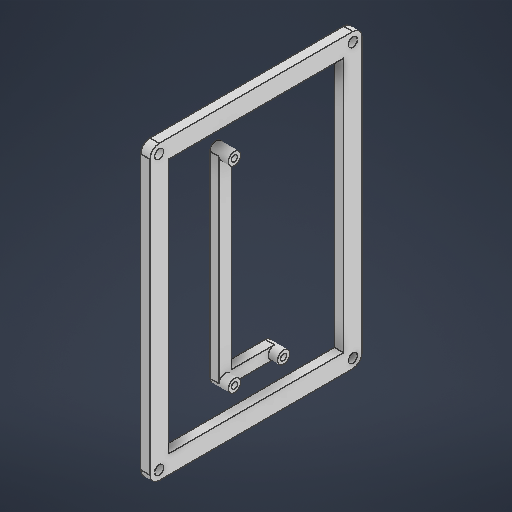
# Autodesk Inventor part: servo_drever_support
Saved by Autodesk Inventor 2026.1 (Build 301233000, 233)
## iProperties
Created: 2026-05-02
Part Number: servo_drever_support
Material: Generic
Document SubType Name: Modeling
Designer: emanuel
Density: 1 g/cm^3
Appearance: Default
Author: emanuel
Autodesk Inventor part; units mm, degrees
ref_plane "YZ Plane" through (0, 0, 0) normal (1, 0, 0) x (0, 1, 0)
ref_plane "XZ Plane" through (0, 0, 0) normal (0, 1, 0) x (-1, 0, 0)
ref_plane "XY Plane" through (0, 0, 0) normal (0, 0, 1) x (1, 0, 0)
sketch "Sketch1" plane through (0, 0, 0) normal (1, 0, 0) x (0, 1, 0)
  line L0 (0, 0) -> (0, -16)
  circle A0 centre (0, 0) radius 1
  circle A1 centre (0, -16) radius 1
  line L1 (0, 0) -> (64, 0)
  circle A2 centre (64, 0) radius 1
  line L2 (64, 0) -> (0, 0) construction
  line L3 (64, 2) -> (0, 2)
  line L4 (0, -2) -> (64, -2)
  arc A3 (64, -2) -> (64, 2) centre (64, 0) ccw
  arc A4 (0, 2) -> (0, -2) centre (0, 0) ccw
  line L5 (0, 0) -> (0, -16) construction
  line L6 (-2, 0) -> (-2, -16)
  line L7 (2, -16) -> (2, 0)
  arc A5 (2, 0) -> (-2, 0) centre (0, 0) ccw
  arc A6 (-2, -16) -> (2, -16) centre (0, -16) ccw
  point P0 (32, 0)
  point P1 (0, -8)
  point P2 (2, -2)
  dimension "d0" = 16
  dimension "d1" = 2
  dimension "d2" = 2
  dimension "d3" = 64
  dimension "d4" = 2
  dimension "d5" = 4
  dimension "d6" = 4
  constraints: 20 end point, 8 point on circle, 8 tangent, 7 centre point, 4 equal length, 3 coincident, 2 midpoint, 1 horizontal, 1 vertical
  measures "d0" distance of L0.start L0.end
  measures "d1" diameter of A0
  measures "d2" diameter of A1
  measures "d3" distance of L1.start L1.end
  measures "d4" diameter of A2
  measures "d5" diameter of A4
  measures "d6" diameter of A6
extrude "Extrusion1" add sketch "Sketch1" along normal blind 3 contours A0 L1 L7 L4 L0 | L0 A4 A5 L1 A0 | L4 L7 A6 L6 A4 | A5 L3 A3 L4 L7
sketch "Sketch2" plane through (3, 0, 0) normal (1, 0, 0) x (0, 0, -1)
  circle A0 centre (0, 64) radius 1 projected
  circle A1 centre (0, 64) radius 1
  circle A2 centre (0, 64) radius 2
  circle A3 centre (0, 0) radius 1
  circle A4 centre (0, 0) radius 2
  circle A5 centre (16, 0) radius 1 projected
  circle A6 centre (16, 0) radius 1
  circle A7 centre (16, 0) radius 2
  dimension "d9" = 2
  dimension "d10" = 4
  dimension "d11" = 2
  dimension "d12" = 4
  constraints: 6 centre point, 6 coincident
  measures "d9" diameter of A3
  measures "d10" diameter of A4
  measures "d11" diameter of A6
  measures "d12" diameter of A7
extrude "Extrusion2" add sketch "Sketch2" along normal blind 3
sketch "Sketch3" plane through (3, 0, 0) normal (1, 0, 0) x (0, 0, -1)
  arc A0 (0, -2) -> (-2, 0) centre (0, 0) ccw projected
  line L0 (0, 0) -> (0, 30)
  line L1 (0, 30) -> (10, 30)
  line L2 (-21.5, 74.5) -> (41.5, 74.5)
  line L3 (41.5, 74.5) -> (41.5, -14.5)
  line L4 (41.5, -14.5) -> (-21.5, -14.5)
  line L5 (-21.5, -14.5) -> (-21.5, 74.5)
  line L6 (-21.5, 74.5) -> (41.5, -14.5) construction
  line L7 (41.5, 74.5) -> (-21.5, -14.5) construction
  circle A1 centre (-21.5, 74.5) radius 1.5
  circle A2 centre (41.5, 74.5) radius 1.5
  circle A3 centre (41.5, -14.5) radius 1.5
  circle A4 centre (-21.5, -14.5) radius 1.5
  line L8 (-21.5, -14.5) -> (41.5, -14.5) construction
  line L9 (-21.5, -17.5) -> (41.5, -17.5)
  line L10 (41.5, -11.5) -> (-21.5, -11.5)
  arc A5 (-21.5, -11.5) -> (-21.5, -17.5) centre (-21.5, -14.5) ccw
  arc A6 (41.5, -17.5) -> (41.5, -11.5) centre (41.5, -14.5) ccw
  line L11 (41.5, -14.5) -> (41.5, 74.5) construction
  line L12 (44.5, -14.5) -> (44.5, 74.5)
  line L13 (38.5, 74.5) -> (38.5, -14.5)
  arc A7 (38.5, -14.5) -> (44.5, -14.5) centre (41.5, -14.5) ccw
  arc A8 (44.5, 74.5) -> (38.5, 74.5) centre (41.5, 74.5) ccw
  line L14 (41.5, 74.5) -> (-21.5, 74.5) construction
  line L15 (41.5, 77.5) -> (-21.5, 77.5)
  line L16 (-21.5, 71.5) -> (41.5, 71.5)
  arc A9 (41.5, 71.5) -> (41.5, 77.5) centre (41.5, 74.5) ccw
  arc A10 (-21.5, 77.5) -> (-21.5, 71.5) centre (-21.5, 74.5) ccw
  line L17 (-21.5, 74.5) -> (-21.5, -14.5) construction
  line L18 (-24.5, 74.5) -> (-24.5, -14.5)
  line L19 (-18.5, -14.5) -> (-18.5, 74.5)
  arc A11 (-18.5, 74.5) -> (-24.5, 74.5) centre (-21.5, 74.5) ccw
  arc A12 (-24.5, -14.5) -> (-18.5, -14.5) centre (-21.5, -14.5) ccw
  point P0 (10, -14.5)
  point P1 (41.5, 30)
  point P2 (10, 74.5)
  point P3 (-21.5, 30)
  point P4 (-18.5, -11.5)
  point P5 (-18.5, 71.5)
  point P6 (38.5, 71.5)
  point P7 (38.5, -11.5)
  dimension "d15" = 30
  dimension "d16" = 10
  dimension "d17" = 63
  dimension "d18" = 89
  dimension "d19" = 3
  dimension "d20" = 3
  dimension "d21" = 3
  dimension "d22" = 3
  dimension "d23" = 6
  dimension "d24" = 6
  dimension "d25" = 6
  dimension "d26" = 6
  constraints: 48 end point, 16 point on circle, 16 tangent, 12 centre point, 8 equal length, 6 midpoint, 4 coincident, 3 perpendicular, 2 horizontal, 1 vertical
  measures "d15" distance of L0.start L0.end
  measures "d16" distance of L0.end L1.end
  measures "d17" distance of L3.end L4.end
  measures "d18" distance of L2.end L3.end
  measures "d19" diameter of A1
  measures "d20" diameter of A2
  measures "d21" diameter of A3
  measures "d22" diameter of A4
  measures "d23" diameter of A6
  measures "d24" diameter of A8
  measures "d25" diameter of A10
  measures "d26" diameter of A12
extrude "Extrusion3" add sketch "Sketch3" against normal blind 3 contours A1 L5 A10 A11 L2 | L2 L19 L16 L5 A1 | A11 L15 A8 L2 | L2 L13 L16 L19 | L16 L19 L10 L5 | L5 A5 L18 A10 | A8 A9 L3 A2 L2 | L2 A2 L3 L16 L13 | L10 L19 L4 A4 L5 | L5 A4 L4 A12 A5 | L16 L3 L10 L13 | L10 L13 L4 L19 | L10 L3 A3 L4 L13 | A9 L12 A6 L3 | L4 A7 L9 A12 | A6 A7 L4 A3 L3
body "Solid1"
